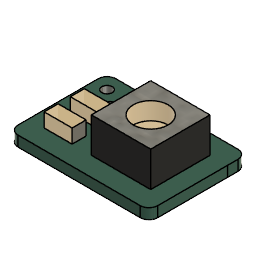
Potentiometer PCB (Autodesk Fusion 360 design; units mm, degrees)
part number: 2026-06-03-23-31-01-197
Autodesk Fusion 360 part; units mm, degrees
note: some values were not read from the file. Set by a fixed rule: which sketch regions a step uses.
sketch "Sketch1" plane through (0, 0, 0) normal (0, 0, 1) x (1, 0, 0)
  line L0 (7, 4.5) -> (7, 0.5)
  line L1 (6.5, 0) -> (0.5, 0)
  arc A0 (6.5, 0) -> (7, 0.5) centre (6.5, 0.5) ccw
  line L2 (0.5, 5.6) -> (6.5, 5.6)
  line L3 (7, 5.1) -> (7, 4.5)
  arc A1 (7, 5.1) -> (6.5, 5.6) centre (6.5, 5.1) ccw
  line L4 (-1, 0.5) -> (-1, 5)
  line L5 (-1, 5) -> (-1, 5.1)
  line L6 (-0.5, 5.6) -> (0.5, 5.6)
  line L7 (-0.5, 0) -> (0.5, 0)
  arc A2 (-0.5, 5.6) -> (-1, 5.1) centre (-0.5, 5.1) ccw
  arc A3 (-1, 0.5) -> (-0.5, 0) centre (-0.5, 0.5) ccw
  constraint tangent L1 A0
  constraint tangent L2 A1
  constraint vertical L4
  constraint tangent L4 A3
  constraint tangent L5 A2
  constraint parallel L4 L5
extrude "Extrude1" add sketch "Sketch1" along normal blind 0.6
sketch "Sketch7" plane through (0, 0, 0.6) normal (0, 0, 1) x (-1, 0, 0)
  line L0 (0.5, 0) -> (-6.5, 0)
  arc A0 (-6.5, 0) -> (-7, -0.5) centre (-6.5, -0.5) ccw
  line L1 (-7, -0.5) -> (-7, -4.5)
  line L2 (-7, -4.5) -> (-7, -5.1)
  arc A1 (-7, -5.1) -> (-6.5, -5.6) centre (-6.5, -5.1) ccw
  line L3 (-6.5, -5.6) -> (0.5, -5.6)
  line L4 (-2.6, -2.8) -> (-2.6, -4.5)
  line L5 (-2.6, -4.5) -> (-6, -4.5)
  line L6 (-6, -4.5) -> (-6, -1.1)
  line L7 (-6, -1.1) -> (-2.6, -1.1)
  line L8 (-2.6, -1.1) -> (-2.6, -2.8)
  line L9 (1, -5.1) -> (1, -0.5)
  arc A2 (1, -0.5) -> (0.5, 0) centre (0.5, -0.5) ccw
  arc A3 (0.5, -5.6) -> (1, -5.1) centre (0.5, -5.1) ccw
  dimension "d30" = 1.7
  dimension "d31" = 3.4
  dimension "d32" = 3.4
  constraint perpendicular L4 L5
  constraint perpendicular L5 L6
  constraint perpendicular L6 L7
  measures "d30" distance of L4.start L4.end
  measures "d31" distance of L4.end L5.end
  measures "d32" distance of L5.end L6.end
extrude "Extrude7" add sketch "Sketch7" along normal blind 2 contours L4 L5 L6 L7 L8
sketch "Sketch8" plane through (0, 0, 2.6) normal (0, 0, 1) x (-1, 0, 0)
  line L0 (-2.6, -1.1) -> (-6, -1.1)
  line L1 (-6, -1.1) -> (-6, -4.5)
  line L2 (-6, -4.5) -> (-2.6, -4.5)
  line L3 (-2.6, -4.5) -> (-2.6, -2.8)
  line L4 (-2.6, -2.8) -> (-2.6, -1.1)
  circle A0 centre (-4.3, -2.8) radius 1
extrude "Extrude8" cut sketch "Sketch8" against normal blind 1 contours A0
sketch "Sketch9" plane through (0, 0, 0.6) normal (0, 0, 1) x (-1, 0, 0)
  line L0 (-2.6, -1.1) -> (-2.6, -2.8)
  line L1 (-2.6, -2.8) -> (-2.6, -4.5)
  line L2 (-2.6, -4.5) -> (-6, -4.5)
  line L3 (-6, -4.5) -> (-6, -1.1)
  line L4 (-6, -1.1) -> (-2.6, -1.1)
  line L5 (-7, -4.5) -> (-7, -5.1)
  arc A0 (-7, -5.1) -> (-6.5, -5.6) centre (-6.5, -5.1) ccw
  line L6 (-6.5, -5.6) -> (0.5, -5.6)
  line L7 (0.5, 0) -> (-6.5, 0)
  arc A1 (-6.5, 0) -> (-7, -0.5) centre (-6.5, -0.5) ccw
  line L8 (-7, -0.5) -> (-7, -4.5)
  line L9 (-1.5, -1.1) -> (0.1, -1.1)
  line L10 (0.1, -1.1) -> (0.1, -1.9)
  line L11 (0.1, -1.9) -> (-1.5, -1.9)
  line L12 (-1.5, -1.9) -> (-1.5, -1.1)
  line L13 (-1.5, -2.6) -> (0.1, -2.6)
  line L14 (0.1, -2.6) -> (0.1, -3.4)
  line L15 (0.1, -3.4) -> (-1.5, -3.4)
  line L16 (-1.5, -3.4) -> (-1.5, -2.6)
  line L17 (1, -5.1) -> (1, -0.5)
  arc A2 (1, -0.5) -> (0.5, 0) centre (0.5, -0.5) ccw
  arc A3 (0.5, -5.6) -> (1, -5.1) centre (0.5, -5.1) ccw
  constraint horizontal L9
  constraint vertical L10
  constraint horizontal L11
  constraint vertical L12
  constraint horizontal L13
  constraint vertical L14
  constraint horizontal L15
  constraint vertical L16
extrude "Extrude9" add sketch "Sketch9" along normal blind 0.8 contours L9 L10 L11 L12 | L13 L14 L15 L16
sketch "Sketch10" plane through (0, 0, 0.6) normal (0, 0, 1) x (-1, 0, 0)
  line L0 (-2.6, -1.1) -> (-2.6, -2.8)
  line L1 (-2.6, -2.8) -> (-2.6, -4.5)
  line L2 (-2.6, -4.5) -> (-6, -4.5)
  line L3 (-6, -4.5) -> (-6, -1.1)
  line L4 (-6, -1.1) -> (-2.6, -1.1)
  line L5 (-7, -4.5) -> (-7, -5.1)
  arc A0 (-7, -5.1) -> (-6.5, -5.6) centre (-6.5, -5.1) ccw
  line L6 (-6.5, -5.6) -> (0.5, -5.6)
  line L7 (0.5, 0) -> (-6.5, 0)
  arc A1 (-6.5, 0) -> (-7, -0.5) centre (-6.5, -0.5) ccw
  line L8 (-7, -0.5) -> (-7, -4.5)
  circle A2 centre (0.2, -4.8) radius 0.3
  circle A3 centre (-1.6, -4.8) radius 0.3
  circle A4 centre (-0.7, -4.1) radius 0.3
  line L9 (-1.5, -1.1) -> (0.1, -1.1)
  line L10 (0.1, -3.4) -> (-1.5, -3.4)
  line L11 (-1.5, -3.4) -> (-1.5, -2.6)
  line L12 (-1.5, -2.6) -> (0.1, -2.6)
  line L13 (0.1, -1.9) -> (-1.5, -1.9)
  line L14 (-1.5, -1.9) -> (-1.5, -1.1)
  line L15 (0.1, -1.1) -> (0.1, -1.9)
  line L16 (0.1, -2.6) -> (0.1, -3.4)
  line L17 (1, -5.1) -> (1, -0.5)
  arc A5 (1, -0.5) -> (0.5, 0) centre (0.5, -0.5) ccw
  arc A6 (0.5, -5.6) -> (1, -5.1) centre (0.5, -5.1) ccw
extrude "Extrude10" cut sketch "Sketch10" against normal blind 0.6 contours A2 | A3 | A4
